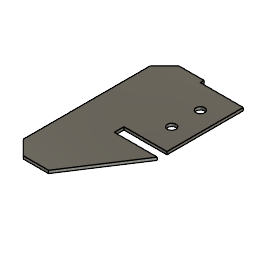
GPL H350 to 200G30_ (Autodesk Fusion 360 design; units mm, degrees)
Autodesk Fusion 360 part; units mm, degrees
sketch "スケッチ1" plane through (0, 0, 0) normal (0, 0, 1) x (1, 0, 0)
  line L0 (-3.5, 163) -> (-86.5, 163)
  line L1 (-86.5, 163) -> (-86.5, -163)
  line L2 (-86.5, -163) -> (-3.5, -163)
  line L3 (86.5, -5) -> (86.5, 155)
  line L4 (82.2546, 155) -> (-86.5, -163) construction
  line L5 (-86.5, 163) -> (46.1223, -86.9125) construction
  line L6 (-3.5, 163) -> (-3.5, 155)
  line L7 (-3.5, 155) -> (86.5, 155)
  line L8 (-86.5, -163) -> (-3.5, -163) construction
  line L9 (-3.5, -163) -> (86.5, -25)
  line L10 (86.5, -25) -> (-3.5, -25)
  line L11 (-3.5, -25) -> (-3.5, -5)
  line L12 (-3.5, -5) -> (86.5, -5)
  dimension "d2" = 326
  dimension "d5" = 83
  dimension "d7" = 90
  dimension "d8" = 20
  constraint horizontal L0
  constraint perpendicular L0 L1
  constraint parallel L0 L2
  constraint parallel L1 L3
  constraint coincident L4 origin
  constraint coincident L5 origin
  constraint vertical L6
  constraint horizontal L7
  constraint coincident L7 L4.start
  constraint perpendicular L1 L8
  constraint coincident L9 L5.end
  constraint horizontal L10
  constraint vertical L11
  constraint horizontal L12
  measures "d2" distance of L0.end L1.end
  measures "d5" distance of L1.end L2.end
  measures "d7" distance of L9.end L10.end
  measures "d8" distance of L9.end L3.start
extrude "押し出し1" add sketch "スケッチ1" along normal blind 6
chamfer "面取り1" distance 30 angle 45 2 edges at (-86.5, -163, 3) (-86.5, 163, 3)
sketch "スケッチ2" plane through (0, 0, 6) normal (0, 0, 1) x (-1, 0, 0)
  line L0 (56.5, -163) -> (86.5, -133)
  line L1 (86.5, -133) -> (86.5, 133)
  line L2 (86.5, 133) -> (56.5, 163)
  line L3 (56.5, 163) -> (3.5, 163)
  line L4 (3.5, 163) -> (-86.5, 25)
  line L5 (-86.5, 25) -> (3.5, 25)
  line L6 (3.5, 25) -> (3.5, 5)
  line L7 (3.5, 5) -> (-86.5, 5)
  line L8 (-86.5, 5) -> (-86.5, -155)
  line L9 (-86.5, -155) -> (3.5, -155)
  line L10 (3.5, -155) -> (3.5, -163)
  line L11 (3.5, -163) -> (56.5, -163)
  line L12 (-86.5, -155) -> (-46.5, -155) construction
  line L13 (-46.5, -155) -> (-46.5, -105) construction
  line L14 (-46.5, -105) -> (-86.5, -105) construction
  line L15 (-86.5, -105) -> (-86.5, -155) construction
  line L16 (-46.5, -105) -> (-46.5, -45) construction
  point P0 (-46.5, -105)
  point P1 (-46.5, -45)
  dimension "d12" = 40
  dimension "d13" = 50
  dimension "d14" = 60
  constraint horizontal L12
  constraint vertical L13
  constraint horizontal L14
  constraint vertical L15
  constraint coincident L8.end L9.start
  constraint perpendicular L14 L16
  constraint coincident P0 L13.end
  constraint coincident P1 L16.end
  measures "d12" distance of L8.end L12.end
  measures "d13" distance of L8.end L14.end
  measures "d14" distance of P0 P1
hole "穴1" at (46.5, 105, 6) at (46.5, 45, 6) direction (0, 0, -1) diameter 18 end through all
equation "d5 = 30 mm + 53 mm"
